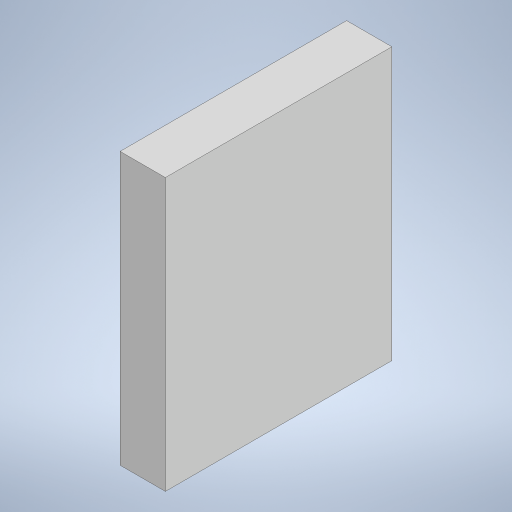
# Autodesk Inventor part: GUIA INTERIOR
Saved by Autodesk Inventor 2023 (Build 270158000, 158)
## iProperties
Created: 2023-03-22
Part Number: GUIA INTERIOR
Material: Generic
Document SubType Name: Modeling
Designer: sebas
Density: 1 g/cm^3
Appearance: Default
Author: sebas
Autodesk Inventor part; units mm, degrees
ref_plane "YZ Plane" through (0, 0, 0) normal (1, 0, 0) x (0, 1, 0)
ref_plane "XZ Plane" through (0, 0, 0) normal (0, 1, 0) x (-1, 0, 0)
ref_plane "XY Plane" through (0, 0, 0) normal (0, 0, 1) x (1, 0, 0)
sketch "Sketch1" plane through (0, 0, 0) normal (0, 1, 0) x (-1, 0, 0)
  line L0 (0, 0) -> (0, -25)
  line L1 (0, -25) -> (-5, -25)
  line L2 (-5, -25) -> (-5, 0)
  line L3 (-5, 0) -> (0, 0)
  dimension "d0" = 25
  dimension "d1" = 5
  dimension "d2" = 25
  dimension "d3" = 5
  constraints: 8 end point, 2 perpendicular, 1 vertical
  measures "d0" distance of L0.start L0.end
  measures "d1" distance of L0.end L1.end
  measures "d2" distance of L1.end L2.end
  measures "d3" distance of L2.end L0.start
extrude "Extrusion1" add sketch "Sketch1" along normal blind 30
body "Solid1"
